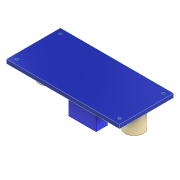
# Autodesk Inventor part: dcdc
Saved by Autodesk Inventor 2022 (Build 260153000, 153)
## iProperties
Created: 2022-11-21
Part Number: dcdc
Material: Generic
Document SubType Name: Modeling
Designer: ferna
Density: 1 g/cm^3
Appearance: Turquoise
Author: ferna
Autodesk Inventor part; units mm, degrees
ref_plane "YZ Plane" through (0, 0, 0) normal (1, 0, 0) x (0, 1, 0)
ref_plane "XZ Plane" through (0, 0, 0) normal (0, 1, 0) x (-1, 0, 0)
ref_plane "XY Plane" through (0, 0, 0) normal (0, 0, 1) x (1, 0, 0)
sketch "Sketch1" plane through (0, 0, 0) normal (0, 1, 0) x (-1, 0, 0)
  line L0 (0, 0) -> (44, 0)
  line L1 (44, 0) -> (44, -21)
  line L2 (44, -21) -> (0, -21)
  line L3 (0, -21) -> (0, 0)
  line L4 (0, 0) -> (0, -2)
  line L5 (0, -2) -> (2, -2)
  circle A0 centre (2, -2) radius 0.51
  line L6 (44, 0) -> (42, 0)
  line L7 (42, 0) -> (42, -2)
  line L8 (44, -21) -> (44, -19)
  line L9 (44, -19) -> (42, -19)
  line L10 (0, -21) -> (0, -19)
  line L11 (0, -19) -> (2, -19)
  circle A1 centre (42, -2) radius 0.51
  circle A2 centre (42, -19) radius 0.51
  circle A3 centre (2, -19) radius 0.51
  dimension "d0" = 44
  dimension "d1" = 21
  dimension "d2" = 2
  dimension "d3" = 2
  dimension "d4" = 1.02
  dimension "d5" = 2
  dimension "d6" = 2
  dimension "d7" = 2
  dimension "d8" = 2
  dimension "d9" = 2
  dimension "d10" = 2
  dimension "d11" = 1.02
  dimension "d12" = 1.02
  dimension "d13" = 1.02
  constraints: 24 end point, 4 centre point, 4 coincident, 4 perpendicular, 4 point on line, 3 parallel, 1 horizontal
  measures "d0" distance of L1.end L2.end
  measures "d1" distance of L0.end L1.end
  measures "d2" distance of L0.start L4.end
  measures "d3" distance of L4.end L5.end
  measures "d4" diameter of A0
  measures "d5" distance of L0.end L6.end
  measures "d6" distance of L6.end L7.end
  measures "d7" distance of L1.end L8.end
  measures "d8" distance of L8.end L9.end
  measures "d9" distance of L2.end L10.end
  measures "d10" distance of L10.end L11.end
  measures "d11" diameter of A1
  measures "d12" diameter of A2
  measures "d13" diameter of A3
extrude "Extrusion1" add sketch "Sketch1" along normal blind 1.524
sketch "Sketch2" plane through (0, 1.524, 0) normal (0, 1, 0) x (1, 0, 0)
  circle A0 centre (-5.1855, 10.8571) radius 3.5384
  circle A1 centre (-38.5669, 10.8571) radius 3.5384
  point P0 (0, 0)
  constraints: 2 centre point
extrude "Extrusion2" add sketch "Sketch2" along normal blind 7.774 separate body
sketch "Sketch3" plane through (0, 0, 0) normal (0, -1, 0) x (1, 0, 0)
  circle A0 centre (-38.5669, -10.8571) radius 3.5384 projected
  circle A1 centre (-5.1855, -10.8571) radius 3.5384 projected
  point P0 (0, 0)
extrude "Extrusion3" add sketch "Sketch3" along normal blind 7.774 separate body
sketch "Sketch4" plane through (-5.1855, 9.298, -10.8571) normal (0, 1, 0) x (1, 0, 0)
  line L0 (6.5142, 3.9863) -> (-37.5817, 3.9863)
  line L1 (-37.5817, 3.9863) -> (-37.5817, -5.5983)
  line L2 (-37.5817, -5.5983) -> (6.5142, -5.5983)
  line L3 (6.5142, -5.5983) -> (6.5142, 3.9863)
  point P0 (5.1855, -10.8571)
  constraints: 8 end point, 2 parallel, 1 horizontal, 1 perpendicular
extrude "Extrusion4" cut sketch "Sketch4" against normal blind 7.774 bodies 2
sketch "Sketch5" plane through (0, 0, 0) normal (0, -1, 0) x (1, 0, 0)
  line L0 (-10.6228, -17.5049) -> (-20.6228, -17.5049)
  line L1 (-20.6228, -17.5049) -> (-20.6228, -7.5049)
  line L2 (-20.6228, -7.5049) -> (-10.6228, -7.5049)
  line L3 (-10.6228, -7.5049) -> (-10.6228, -17.5049)
  point P0 (0, 0)
  dimension "d22" = 10
  dimension "d23" = 10
  constraints: 8 end point, 2 parallel, 1 horizontal, 1 perpendicular
  measures "d22" distance of L1.end L2.end
  measures "d23" distance of L0.end L1.end
extrude "Extrusion5" add sketch "Sketch5" along normal blind 5 separate body
sketch "Sketch6" plane through (0, 0, 0) normal (0, -1, 0) x (1, 0, 0)
  line L0 (-10.6495, -5.9119) -> (-21.2585, -5.9119)
  line L1 (-21.2585, -5.9119) -> (-21.2585, -1.5387)
  line L2 (-21.2585, -1.5387) -> (-10.6495, -1.5387)
  line L3 (-10.6495, -1.5387) -> (-10.6495, -5.9119)
  point P0 (0, 0)
  constraints: 8 end point, 2 parallel, 1 horizontal, 1 perpendicular
extrude "Extrusion6" add sketch "Sketch6" along normal blind 7.024 separate body
sketch "Sketch7" plane through (0, 0, 0) normal (0, -1, 0) x (1, 0, 0)
  line L0 (-32.0595, -13.4531) -> (-22.8861, -13.4531)
  line L1 (-22.8861, -13.4531) -> (-22.8861, -6.4315)
  line L2 (-22.8861, -6.4315) -> (-32.0595, -6.4315)
  line L3 (-32.0595, -6.4315) -> (-32.0595, -13.4531)
  point P0 (0, 0)
  constraints: 8 end point, 2 parallel, 1 horizontal, 1 perpendicular
extrude "Extrusion7" add sketch "Sketch7" along normal blind 3 separate body
sketch "Sketch8" plane through (0, 0, 0) normal (0, -1, 0) x (1, 0, 0)
  line L0 (-32.0595, -13.4531) -> (-22.8861, -13.4531) projected
  line L1 (-31.301, -13.4531) -> (-30.0033, -13.4531)
  line L2 (-30.0033, -13.4531) -> (-30.0033, -14.2432)
  line L3 (-30.0033, -14.2432) -> (-31.301, -14.2432)
  line L4 (-31.301, -14.2432) -> (-31.301, -13.4531)
  line L5 (-29.301, -13.4531) -> (-28.0033, -13.4531)
  line L6 (-28.0033, -13.4531) -> (-28.0033, -14.2432)
  line L7 (-28.0033, -14.2432) -> (-29.301, -14.2432)
  line L8 (-29.301, -14.2432) -> (-29.301, -13.4531)
  line L9 (-27.301, -13.4531) -> (-26.0033, -13.4531)
  line L10 (-26.0033, -13.4531) -> (-26.0033, -14.2432)
  line L11 (-26.0033, -14.2432) -> (-27.301, -14.2432)
  line L12 (-27.301, -14.2432) -> (-27.301, -13.4531)
  line L13 (-25.301, -13.4531) -> (-24.0033, -13.4531)
  line L14 (-24.0033, -13.4531) -> (-24.0033, -14.2432)
  line L15 (-24.0033, -14.2432) -> (-25.301, -14.2432)
  line L16 (-25.301, -14.2432) -> (-25.301, -13.4531)
  line L17 (-31.301, -5.6541) -> (-30.0033, -5.6541)
  line L18 (-30.0033, -5.6541) -> (-30.0033, -6.4442)
  line L19 (-30.0033, -6.4442) -> (-31.301, -6.4442)
  line L20 (-31.301, -6.4442) -> (-31.301, -5.6541)
  line L21 (-29.301, -5.6541) -> (-28.0033, -5.6541)
  line L22 (-28.0033, -5.6541) -> (-28.0033, -6.4442)
  line L23 (-28.0033, -6.4442) -> (-29.301, -6.4442)
  line L24 (-29.301, -6.4442) -> (-29.301, -5.6541)
  line L25 (-27.301, -5.6541) -> (-26.0033, -5.6541)
  line L26 (-26.0033, -5.6541) -> (-26.0033, -6.4442)
  line L27 (-26.0033, -6.4442) -> (-27.301, -6.4442)
  line L28 (-27.301, -6.4442) -> (-27.301, -5.6541)
  line L29 (-25.301, -5.6541) -> (-24.0033, -5.6541)
  line L30 (-24.0033, -5.6541) -> (-24.0033, -6.4442)
  line L31 (-24.0033, -6.4442) -> (-25.301, -6.4442)
  line L32 (-25.301, -6.4442) -> (-25.301, -5.6541)
  point P0 (0, 0)
  dimension "d32" = 2
  dimension "d35" = 7.799
  constraints: 64 end point, 2 horizontal, 2 parallel, 1 collinear, 1 perpendicular, 1 point on line, 1 vertical, 55 other
  measures "d32" distance of L1.start L5.start
  measures "d35" distance of L1.start L17.start
extrude "Extrusion8" add sketch "Sketch8" along normal blind 2 separate body
body "Solid1"
body "Solid2"
body "Solid3"
body "Solid4"
body "Solid5"
body "Solid6"
body "Solid7"
